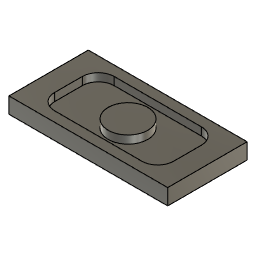
Day #13 Pcoket 5mm Milling v1 (Autodesk Fusion 360 design; units mm, degrees)
Autodesk Fusion 360 part; units mm, degrees
sketch "Sketch1" plane through (0, 0, 0) normal (0, 0, 1) x (1, 0, 0)
  line L0 (-100, 50) -> (100, 50)
  line L1 (100, 50) -> (100, -50)
  line L2 (100, -50) -> (-100, -50)
  line L3 (-100, -50) -> (-100, 50)
  line L4 (-100, 50) -> (100, -50) construction
  line L5 (100, 50) -> (-100, -50) construction
  line L6 (-55, 37.5) -> (55, 37.5)
  line L7 (75, 17.5) -> (75, -17.5)
  line L8 (55, -37.5) -> (-55, -37.5)
  line L9 (-75, -17.5) -> (-75, 17.5)
  line L10 (-75, 37.5) -> (75, -37.5) construction
  line L11 (75, 37.5) -> (-75, -37.5) construction
  arc A0 (-55, 37.5) -> (-75, 17.5) centre (-55, 17.5) ccw
  arc A1 (-75, -17.5) -> (-55, -37.5) centre (-55, -17.5) ccw
  arc A2 (55, -37.5) -> (75, -17.5) centre (55, -17.5) ccw
  arc A3 (75, 17.5) -> (55, 37.5) centre (55, 17.5) ccw
  circle A4 centre (0, 0) radius 25
  dimension "d1" = 200
  dimension "d2" = 100
  dimension "d3" = 150
  dimension "d4" = 75
  dimension "d5" = 20
  dimension "d6" = 20
  dimension "d7" = 50
  constraint horizontal L0
  constraint perpendicular L0 L1
  constraint parallel L0 L2
  constraint parallel L1 L3
  constraint coincident L4 A4.centre
  constraint coincident L5 A4.centre
  constraint coincident A4.centre origin
  constraint horizontal L6
  constraint perpendicular L6 L7
  constraint parallel L6 L8
  constraint parallel L7 L9
  constraint coincident L10 A4.centre
  constraint coincident L11 A4.centre
  constraint coincident L10.start L9
  constraint coincident L10.start L6
  constraint tangent L9 A0
  constraint tangent L6 A0
  constraint coincident L11.end L9
  constraint coincident L11.end L8
  constraint tangent L9 A1
  constraint tangent L8 A1
  constraint coincident L10.end L8
  constraint coincident L10.end L7
  constraint tangent L8 A2
  constraint tangent L7 A2
  constraint equal A1 A2
  constraint coincident L11.start L6
  constraint coincident L11.start L7
  constraint tangent L6 A3
  constraint tangent L7 A3
  constraint equal A1 A3
  measures "d1" distance of L1.end L2.end
  measures "d2" distance of L0.end L1.end
  measures "d3" distance of L10.end L11.end
  measures "d4" distance of L11.start L10.end
  measures "d5" radius of A0
  measures "d6" radius of A1
  measures "d7" diameter of A4
extrude "Extrude1" add sketch "Sketch1" along normal blind 20 contours L0 L1 L2 L3
extrude "Extrude2" add sketch "Sketch1" along normal blind 10 contours L6 L7 L8 L9 A0 A1 A2 A3
extrude "Extrude3" add sketch "Sketch1" along normal blind 20 contours A4
